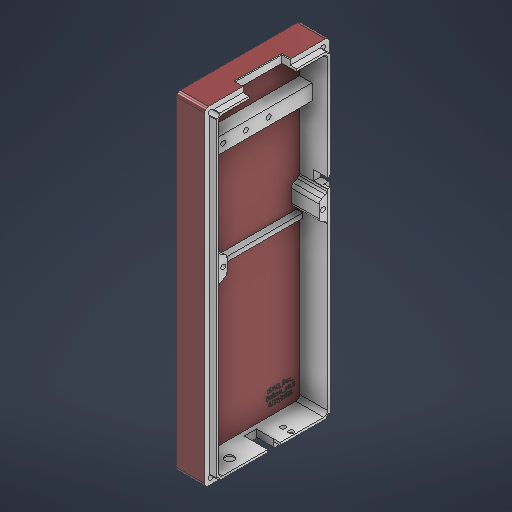
# Autodesk Inventor part: cDAQ_Box_Bottom_v0.2
Saved by Autodesk Inventor 2027 (Build 310192000, 192)
## iProperties
Created: 2026-05-08
Part Number: cDAQ_Box_Bottom_v0.2
Material: Generic
Document SubType Name: Modeling
Designer: giese
Density: 1 g/cm^3
Appearance: Default
Author: giese
Autodesk Inventor part; units mm, degrees
(part 1 of 2)
ref_plane "YZ Plane" through (0, 0, 0) normal (1, 0, 0) x (0, 1, 0)
ref_plane "XZ Plane" through (0, 0, 0) normal (0, 1, 0) x (-1, 0, 0)
ref_plane "XY Plane" through (0, 0, 0) normal (0, 0, 1) x (1, 0, 0)
sketch "Sketch1" plane through (0, 0, 0) normal (1, 0, 0) x (0, 1, 0)
  line L0 (37.5698, 53.1667) -> (-230.1462, 53.1667)
  line L1 (-230.1462, 53.1667) -> (-230.1462, -48.4333)
  line L2 (-230.1462, -48.4333) -> (37.5698, -48.4333)
  line L3 (37.5698, -48.4333) -> (37.5698, 53.1667)
  point P0 (0, 0)
  dimension "d0" = 101.6
  dimension "d1" = 267.716
  constraints: 8 end point, 2 parallel, 1 horizontal, 1 perpendicular
  measures "d0" distance of L2.end L0.start
  measures "d1" distance of L1.end L2.end
extrude "Extrusion1" add sketch "Sketch1" along normal blind 22.86
sketch "Sketch2" plane through (22.86, 0, 0) normal (1, 0, 0) x (0, 0, -1)
  line L0 (42.0833, 31.2198) -> (-46.8167, 31.2198)
  line L1 (-46.8167, 31.2198) -> (-46.8167, -223.7962)
  line L2 (-46.8167, -223.7962) -> (42.0833, -223.7962)
  line L3 (42.0833, -223.7962) -> (42.0833, 31.2198)
  line L4 (48.4333, 37.5698) -> (-53.1667, 37.5698) projected
  line L5 (-53.1667, 37.5698) -> (-53.1667, -230.1462) projected
  line L6 (-53.1667, -230.1462) -> (48.4333, -230.1462) projected
  point P0 (0, 0)
  dimension "d4" = 255.016
  dimension "d5" = 88.9
  dimension "d8" = 6.35
  dimension "d21" = 6.35
  dimension "d690" = 6.35
  constraints: 8 end point, 2 parallel, 1 horizontal, 1 perpendicular
  measures "d4" distance of L2.end L0.start
  measures "d5" distance of L0.start L0.end
  measures "d8" distance between parallel lines of L0 L4
  measures "d21" distance between parallel lines of L5 L1
  measures "d690" distance between parallel lines of L6 L2
extrude "Extrusion2" cut sketch "Sketch2" against normal blind 17.78
sketch "Sketch3" plane through (0, 0, 0) normal (-1, 0, 0) x (0, 0, 1)
  circle A0 centre (-6.6909, -2.0542) radius 2
  circle A1 centre (11.8079, -2.0542) radius 2
  circle A2 centre (30.3067, -2.0542) radius 2
  line L0 (-48.4333, -230.1462) -> (-48.4333, 37.5698) projected
  line L1 (-48.4333, 37.5698) -> (53.1667, 37.5698) projected
  line L2 (53.1667, 37.5698) -> (53.1667, -230.1462) projected
  line L3 (46.8167, 31.2198) -> (-42.0833, 31.2198) projected
  point P0 (0, 0)
  point P1 (-0.896, -23.7433)
  point P2 (-45.1848, 27.0137)
  dimension "d9" = 18.4988
  dimension "d10" = 4
  dimension "d11" = 4
  dimension "d12" = 18.4988
  dimension "d13" = 36.9976
  dimension "d18" = 22.86
  dimension "d22" = 4
  dimension "d58" = 39.624
  constraints: 3 centre point
  measures "d9" distance of A0.centre A1.centre
  measures "d10" diameter of A1
  measures "d11" diameter of A2
  measures "d12" distance of A1.centre A2.centre
  measures "d13" distance of A0.centre A2.centre
  measures "d18" distance from line of L2 A2.centre
  measures "d22" diameter of A0
  measures "d58" distance from line of L1 A2.centre
extrude "Extrusion3" cut sketch "Sketch3" against normal blind 5.08
sketch "Sketch5" plane through (0, -230.1462, -48.4333) normal (0, 0, -1) x (-1, 0, 0)
  line L0 (-27.2034, 165.862) -> (-16.51, 165.862)
  line L1 (-16.51, 165.862) -> (-16.51, 173.862)
  line L2 (-16.51, 173.862) -> (-27.2034, 173.862)
  line L3 (-27.2034, 173.862) -> (-27.2034, 165.862)
  line L4 (0, 267.716) -> (-22.86, 267.716) projected
  line L5 (0, 0) -> (0, 267.716) projected
  line L6 (-22.86, 0) -> (-22.86, 267.716) projected
  point P0 (0, 230.1462)
  point P1 (-21.8567, 173.862)
  point P2 (-21.8567, 165.862)
  dimension "d28" = 10.6934
  dimension "d30" = 8
  dimension "d31" = 16.51
  dimension "d34" = 101.854
  dimension "d215" = 4.3434
  constraints: 8 end point, 2 midpoint, 2 parallel, 1 horizontal, 1 perpendicular
  measures "d28" distance between parallel lines of L1 L3
  measures "d30" distance of point (-21.857, 173.862) point (-21.857, 165.862)
  measures "d31" distance between parallel lines of L5 L1
  measures "d34" distance between parallel lines of L4 L0
  measures "d215" distance between parallel lines of L6 L3
extrude "Extrusion4" cut sketch "Sketch5" against normal blind 24.13
sketch "Sketch6" plane through (0, -230.1462, -48.4333) normal (0, -1, 0) x (1, 0, 0)
  line L0 (24.08, 55.136) -> (16.08, 55.136)
  line L1 (16.08, 45.136) -> (24.08, 45.136)
  line L2 (0, 101.6) -> (0, 0) projected
  line L3 (28.36, 53.1359) -> (28.36, 47.136)
  line L4 (24.08, 55.136) -> (28.36, 53.1359)
  line L5 (28.36, 47.136) -> (24.08, 45.136)
  line L6 (0, 0) -> (22.86, 0) projected
  line L7 (22.86, 95.25) -> (22.86, 6.35) projected
  line L8 (22.86, 41.9134) -> (22.86, 37.4697)
  line L9 (16.08, 55.136) -> (8.636, 55.136)
  line L10 (8.636, 55.136) -> (8.636, 45.136)
  line L11 (8.636, 45.136) -> (21.16, 45.136)
  point P0 (0, 48.4333)
  point P1 (20.08, 55.136)
  point P2 (20.08, 45.136)
  point P3 (16.08, 50.136)
  dimension "d39" = 6
  dimension "d48" = 55.136
  dimension "d221" = 0
  dimension "d223" = 2
  dimension "d224" = 2
  dimension "d225" = 5.5
  dimension "d227" = 4.28
  dimension "d672" = 8.636
  constraints: 18 end point, 2 horizontal, 2 midpoint, 2 parallel, 2 point on line, 1 perpendicular, 1 vertical
  measures "d39" distance of L3.start L3.end
  measures "d48" distance between parallel lines of L6 L0
  measures "d221" horizontal distance of L0.start L1.end
  measures "d223" vertical distance of L3.end L1.end
  measures "d224" vertical distance of L0.start L3.start
  measures "d225" distance between parallel lines of L3 L7
  measures "d227" distance from line of L1.end L3
  measures "d672" distance between parallel lines of L2 L10
extrude "Extrusion5" cut sketch "Sketch6" against normal blind 6.35
sketch "Sketch7" plane through (0, 37.5698, 53.1667) normal (0, 1, 0) x (1, 0, 0)
  line L0 (31.0134, 69.85) -> (16.002, 69.85)
  line L1 (16.002, 69.85) -> (16.002, 31.75)
  line L2 (16.002, 31.75) -> (31.0134, 31.75)
  line L3 (31.0134, 31.75) -> (31.0134, 69.85)
  line L4 (0, 0) -> (22.86, 0) projected
  line L5 (0, 101.6) -> (0, 0) projected
  line L6 (22.86, 101.6) -> (22.86, 0) projected
  point P0 (0, 53.1667)
  point P1 (22.86, 69.85)
  point P2 (22.86, 31.75)
  dimension "d51" = 38.1
  dimension "d52" = 31.75
  dimension "d55" = 16.002
  dimension "d56" = 15.0114
  dimension "d57" = 8.1534
  constraints: 8 end point, 2 parallel, 1 horizontal, 1 perpendicular
  measures "d51" distance of L2.end L0.start
  measures "d52" distance between parallel lines of L4 L2
  measures "d55" distance between parallel lines of L5 L1
  measures "d56" distance between parallel lines of L3 L1
  measures "d57" distance between parallel lines of L6 L3
extrude "Extrusion6" cut sketch "Sketch7" against normal blind 7.62
fillet "Fillet1" radius 3.175 4 edges at (11.43, 37.5698, -48.4333) (11.43, 37.5698, 53.1667) (11.43, -230.1462, -48.4333) (11.43, -230.1462, 53.1667)
sketch "Sketch8" plane through (0, 0, 0) normal (-1, 0, 0) x (0, 0, 1)
  line L0 (-8.4625, -5.5848) -> (-4.9319, -5.5848)
  line L1 (-8.4625, 1.4764) -> (-4.9319, 1.4764)
  line L2 (-8.4625, -5.5848) -> (-10.5009, -2.0542)
  line L3 (-8.4625, 1.4764) -> (-10.5009, -2.0542)
  line L4 (-4.9319, -5.5848) -> (-2.8936, -2.0542)
  line L5 (-4.9319, 1.4764) -> (-2.8936, -2.0542)
  circle A0 centre (-6.6909, -2.0542) radius 2 projected
  line L6 (10.0363, -5.5848) -> (13.5669, -5.5848)
  line L7 (10.0363, 1.4764) -> (13.5669, 1.4764)
  line L8 (10.0363, -5.5848) -> (7.9979, -2.0542)
  line L9 (10.0363, 1.4764) -> (7.9979, -2.0542)
  line L10 (13.5669, -5.5848) -> (15.6053, -2.0542)
  line L11 (13.5669, 1.4764) -> (15.6053, -2.0542)
  circle A1 centre (11.8079, -2.0542) radius 2 projected
  line L12 (28.5351, -5.5848) -> (26.4967, -2.0542)
  line L13 (28.5351, 1.4764) -> (26.4967, -2.0542)
  line L14 (28.5351, -5.5848) -> (32.0657, -5.5848)
  line L15 (28.5351, 1.4764) -> (32.0657, 1.4764)
  line L16 (32.0657, -5.5848) -> (34.1041, -2.0542)
  line L17 (32.0657, 1.4764) -> (34.1041, -2.0542)
  circle A2 centre (30.3067, -2.0542) radius 2 projected
  point P0 (-6.6972, -5.5848)
  point P1 (11.8016, -5.5848)
  point P2 (30.3004, -5.5848)
  point P3 (-10.5009, -2.0542)
  point P4 (-2.8936, -2.0542)
  point P5 (15.6053, -2.0542)
  point P6 (7.9979, -2.0542)
  point P7 (34.1041, -2.0542)
  point P8 (26.4967, -2.0542)
  dimension "d60" = 7.0612
  dimension "d61" = 120
  dimension "d62" = 120
  dimension "d63" = 120
  dimension "d64" = 120
  dimension "d65" = 3.5306
  dimension "d66" = 3.5306
  dimension "d67" = 3.5306
  dimension "d68" = 3.5306
  dimension "d69" = 3.5306
  dimension "d70" = 3.5306
  dimension "d71" = 0
  dimension "d72" = 7.6074
  dimension "d73" = 3.81
  dimension "d74" = 0
  dimension "d75" = 7.0612
  dimension "d76" = 120
  dimension "d77" = 120
  dimension "d78" = 120
  dimension "d79" = 120
  dimension "d80" = 3.5306
  dimension "d81" = 3.5306
  dimension "d82" = 3.5306
  dimension "d83" = 3.5306
  dimension "d84" = 3.5306
  dimension "d85" = 3.5306
  dimension "d86" = 0
  dimension "d87" = 7.6074
  dimension "d91" = 0
  dimension "d92" = 3.81
  dimension "d93" = 7.0612
  dimension "d94" = 120
  dimension "d95" = 120
  dimension "d96" = 120
  dimension "d97" = 120
  dimension "d98" = 3.5306
  dimension "d99" = 3.5306
  dimension "d100" = 3.5306
  dimension "d101" = 3.5306
  dimension "d102" = 3.5306
  dimension "d103" = 3.5306
  dimension "d104" = 0
  dimension "d105" = 7.6074
  dimension "d108" = 0
  dimension "d109" = 3.81
  constraints: 36 end point, 6 horizontal, 3 midpoint
  measures "d60" distance from line of point (-6.697, -5.585) L1
  measures "d61" angle of L0 L2
  measures "d62" angle of L1 L3
  measures "d63" angle of L4 L0
  measures "d64" angle of L5 L1
  measures "d65" distance of L0.start L0.end
  measures "d66" distance of L1.start L1.end
  measures "d67" vertical distance of L1.start L3.end
  measures "d68" vertical distance of L0.start L2.end
  measures "d69" vertical distance of L1.end L5.end
  measures "d70" vertical distance of L0.end L4.end
  measures "d71" horizontal distance of L0.start L1.start
  measures "d72" distance of L4.end L2.end
  measures "d73" distance of A0.centre L2.end
  measures "d74" vertical distance of A0.centre L4.end
  measures "d75" distance from line of point (11.802, -5.585) L7
  measures "d76" angle of L6 L8
  measures "d77" angle of L7 L9
  measures "d78" angle of L10 L6
  measures "d79" angle of L11 L7
  measures "d80" distance of L8.start L6.end
  measures "d81" distance of L9.start L7.end
  measures "d82" vertical distance of L9.start L9.end
  measures "d83" vertical distance of L8.start L8.end
  measures "d84" vertical distance of L7.end L11.end
  measures "d85" vertical distance of L6.end L10.end
  measures "d86" horizontal distance of L8.start L9.start
  measures "d87" distance of L10.end L8.end
  measures "d91" vertical distance of A1.centre L8.end
  measures "d92" distance of A1.centre L8.end
  measures "d93" distance from line of point (30.3, -5.585) L15
  measures "d94" angle of L14 L12
  measures "d95" angle of L15 L13
  measures "d96" angle of L16 L14
  measures "d97" angle of L17 L15
  measures "d98" distance of L12.start L16.start
  measures "d99" distance of L15.start L15.end
  measures "d100" vertical distance of L15.start L13.end
  measures "d101" vertical distance of L12.start L12.end
  measures "d102" vertical distance of L15.end L17.end
  measures "d103" vertical distance of L16.start L16.end
  measures "d104" horizontal distance of L12.start L15.start
  measures "d105" distance of L16.end L12.end
  measures "d108" vertical distance of A2.centre L12.end
  measures "d109" distance of A2.centre L12.end
extrude "Extrusion7" cut sketch "Sketch8" against normal blind 4 contours L2 L3 L1 L5 L4 L0 | A0 | L8 L9 L7 L11 L10 L6 | A1 | L12 L13 L15 L17 L16 L14 | A2
sketch "Sketch9" plane through (5.08, 0, 0) normal (1, 0, 0) x (0, 0, -1)
  arc A0 (24.8089, -180.8044) -> (19.3527, -180.8044) centre (22.0808, -178.3302) ccw
  line L0 (45.2583, 37.5698) -> (16.6833, 37.5698) projected
  line L1 (42.0833, 31.2198) -> (42.0833, -223.7962) projected
  arc A1 (20.1758, -185.9502) -> (23.9858, -185.9502) centre (22.0808, -185.9502) ccw
  line L2 (23.9858, -185.9502) -> (23.9858, -182.9374)
  line L3 (20.1758, -185.9502) -> (20.1758, -182.9374)
  arc A2 (24.8089, -180.8044) -> (23.9858, -182.9374) centre (27.1608, -182.9374) ccw
  arc A3 (20.1758, -182.9374) -> (19.3527, -180.8044) centre (17.0008, -182.9374) ccw
  arc A4 (-25.9911, -180.8044) -> (-31.4473, -180.8045) centre (-28.7192, -178.3302) ccw
  arc A5 (-30.6242, -185.9366) -> (-26.8142, -185.9502) centre (-28.7192, -185.9502) ccw
  line L4 (-26.8142, -185.9502) -> (-26.8142, -182.9374)
  line L5 (-30.6242, -185.9366) -> (-30.6242, -182.9374)
  arc A6 (-25.9911, -180.8044) -> (-26.8142, -182.9374) centre (-23.6392, -182.9374) ccw
  arc A7 (-30.6242, -182.9374) -> (-31.4473, -180.8045) centre (-33.7992, -182.9374) ccw
  line L6 (-21.4167, 37.5698) -> (-49.9917, 37.5698) projected
  line L7 (-46.8167, -223.7962) -> (-46.8167, 31.2198) projected
  point P0 (0, 0)
  point P1 (23.9858, -181.4823)
  point P2 (20.1758, -181.4823)
  point P3 (-26.8142, -181.4823)
  point P4 (-30.6242, -181.4823)
  dimension "d112" = 215.9
  dimension "d114" = 7.366
  dimension "d116" = 3.81
  dimension "d117" = 223.52
  dimension "d118" = 3.175
  dimension "d119" = 7.366
  dimension "d120" = 3.81
  dimension "d121" = 3.175
  dimension "d122" = 215.9
  dimension "d123" = 223.52
  dimension "d125" = 0
  dimension "d128" = 50.8
  dimension "d129" = 20.0025
  dimension "d130" = 0
  constraints: 20 point on circle, 8 centre point, 8 end point, 8 tangent, 4 point on line, 2 equal radius, 2 parallel, 2 vertical
  measures "d112" distance from line of L0 A0.centre
  measures "d114" diameter of A0
  measures "d116" diameter of A1
  measures "d117" distance from line of L0 A1.centre
  measures "d118" radius of A2
  measures "d119" diameter of A4
  measures "d120" diameter of A5
  measures "d121" radius of A6
  measures "d122" distance from line of A4.centre L6
  measures "d123" distance from line of L6 A5.centre
  measures "d125" horizontal distance of A5.centre A4.centre
  measures "d128" distance of A5.centre A1.centre
  measures "d129" distance from line of L1 A0.centre
  measures "d130" horizontal distance of A0.centre A1.centre
extrude "Extrusion8" [suppressed]
sketch "Sketch10" plane through (22.86, 0, 0) normal (1, 0, 0) x (0, 0, -1)
  line L0 (-46.8167, 31.2198) -> (42.0833, 31.2198) projected
  line L1 (-46.8167, 31.2198) -> (42.0833, 31.2198)
  line L2 (42.0833, 33.2264) -> (-46.8167, 33.2264)
  line L3 (-46.8167, 33.2264) -> (-48.8233, 33.2264)
  line L4 (-48.8233, 33.2264) -> (-48.8233, -225.8028)
  line L5 (-48.8233, -225.8028) -> (44.0899, -225.8028)
  line L6 (44.0899, -225.8028) -> (44.0899, 33.2264)
  line L7 (44.0899, 33.2264) -> (41.9392, 33.2264)
  line L8 (42.0833, 31.2198) -> (42.0833, -223.7962) projected
  line L9 (-46.8167, -223.7962) -> (-46.8167, 31.2198) projected
  line L10 (42.0833, -223.7962) -> (-46.8167, -223.7962) projected
  line L11 (45.2583, 37.5698) -> (16.6833, 37.5698) projected
  dimension "d202" = 2.0066
  dimension "d203" = 2.0066
  dimension "d204" = 2.0066
  dimension "d205" = 2.0066
  dimension "d208" = 4.3434
  constraints: 14 end point, 3 perpendicular, 3 point on line, 1 collinear, 1 horizontal
  measures "d202" distance between parallel lines of L0 L2
  measures "d203" distance between parallel lines of L6 L8
  measures "d204" distance between parallel lines of L4 L9
  measures "d205" distance between parallel lines of L5 L10
  measures "d208" distance between parallel lines of L11 L2
extrude "Extrusion9" add sketch "Sketch10" along normal blind 5
fillet "Fillet2" radius 3.175 8 edges at (16.47, 31.2198, -42.0833) (16.47, 31.2198, 46.8167) (16.47, -223.7962, 46.8167) (16.47, -223.7962, -42.0833) (25.36, 33.2264, -44.0899) (25.36, 33.2264, 48.8233) (25.36, -225.8028, -44.0899) (25.36, -225.8028, 48.8233)
sketch "Sketch13" plane through (27.86, 0, 0) normal (1, 0, 0) x (0, 0, -1)
  arc A0 (44.0833, 30.0448) -> (40.9083, 33.2198) centre (40.9083, 30.0448) ccw projected
  arc A1 (-45.6417, 33.2198) -> (-48.8167, 30.0448) centre (-45.6417, 30.0448) ccw projected
  arc A2 (40.9083, -212.0802) -> (44.0833, -208.9052) centre (40.9083, -208.9052) ccw projected
  arc A3 (-48.8167, -208.9052) -> (-45.6417, -212.0802) centre (-45.6417, -208.9052) ccw projected
  line L0 (-21.4167, 37.5698) -> (-49.9917, 37.5698) projected
  line L1 (-53.1667, 34.3948) -> (-53.1667, -226.9712) projected
  line L2 (-49.9917, -230.1462) -> (45.2583, -230.1462) projected
  arc A4 (-48.8167, -208.9052) -> (-45.6417, -212.0802) centre (-45.6417, -208.9052) ccw projected
  circle A5 centre (-48.0867, -225.0662) radius 1.9939
  circle A6 centre (43.3533, -225.0662) radius 1.9939
  line L3 (48.4333, -226.9712) -> (48.4333, 34.3948) projected
  circle A7 centre (43.3533, 32.4898) radius 1.9939
  line L4 (45.2583, 37.5698) -> (16.6833, 37.5698) projected
  circle A8 centre (-48.0867, 32.4898) radius 1.9939
  arc A9 (41.4904, -28.6131) -> (38.3154, -25.4381) centre (38.3154, -28.6131) ccw
  circle A10 centre (38.2733, -76.7302) radius 1.9939
  circle A11 centre (-43.0067, -76.7302) radius 1.9939
  point P0 (0, 0)
  point P1 (-47.8868, 32.2898)
  point P2 (-47.8868, -211.1503)
  point P3 (-47.8868, -211.1503)
  point P4 (45.8404, -24.2631)
  point P5 (42.6654, -21.0881)
  dimension "d405" = 120
  dimension "d178" = 5.08
  dimension "d179" = 5.08
  dimension "d180" = 3.9878
  dimension "d181" = 5.08
  dimension "d182" = 5.08
  dimension "d183" = 3.9878
  dimension "d184" = 3.9878
  dimension "d185" = 5.08
  dimension "d186" = 5.08
  dimension "d187" = 3.9878
  dimension "d188" = 5.08
  dimension "d189" = 5.08
  dimension "d326" = 3.9878
  dimension "d327" = 10.16
  dimension "d328" = 114.3
  dimension "d329" = 3.9878
  dimension "d330" = 10.16
  dimension "d331" = 114.3
  constraints: 7 centre point, 5 point on circle
  measures "d178" distance from line of L1 A5.centre
  measures "d179" distance from line of L2 A5.centre
  measures "d180" diameter of A5
  measures "d181" distance from line of L2 A6.centre
  measures "d182" distance from line of L3 A6.centre
  measures "d183" diameter of A6
  measures "d184" diameter of A7
  measures "d185" distance from line of L3 A7.centre
  measures "d186" distance from line of L4 A7.centre
  measures "d187" diameter of A8
  measures "d188" distance from line of L0 A8.centre
  measures "d189" distance from line of L1 A8.centre
  measures "d326" diameter of A10
  measures "d327" distance from line of L3 A10.centre
  measures "d328" distance from line of A10.centre L4
  measures "d329" diameter of A11
  measures "d330" distance from line of L1 A11.centre
  measures "d331" distance from line of L0 A11.centre
extrude "Extrusion11" cut sketch "Sketch13" against normal blind 25.4
sketch "Sketch14" plane through (5.08, 0, 0) normal (1, 0, 0) x (0, 0, -1)
  line L0 (16.7951, -204.0653) -> (36.0118, -204.0653) construction
  line L1 (36.0118, -204.0653) -> (36.0118, -212.8579) construction
  line L2 (36.0118, -212.8579) -> (16.7951, -212.8579) construction
  line L3 (16.7951, -212.8579) -> (16.7951, -204.0653) construction
  spline S0 degree 2 poles (16.7333, -207.2294) (16.4962, -207.2294) (16.1034, -207.0837) (15.9627, -206.9355) knots 0 0 0 1 2 2 2
  spline S1 degree 2 poles (15.9627, -206.9355) (15.8219, -206.7897) (15.6663, -206.3402) (15.6663, -206.0388) knots 0 0 0 1 2 2 2
  spline S2 degree 2 poles (15.6663, -206.0388) (15.6663, -205.7375) (15.8268, -205.2978) (15.9627, -205.1496) knots 0 0 0 1 2 2 2
  spline S3 degree 2 poles (15.9627, -205.1496) (16.0985, -204.999) (16.5011, -204.8384) (16.7333, -204.8384) knots 0 0 0 1 2 2 2
  spline S4 degree 2 poles (16.7333, -204.8384) (16.921, -204.8384) (17.2718, -204.9446) (17.4076, -205.0138) knots 0 0 0 1 2 2 2
  line L4 (17.4076, -205.0138) -> (17.4076, -205.446)
  line L5 (17.4076, -205.446) -> (17.3854, -205.446)
  spline S5 degree 2 poles (17.3854, -205.446) (17.3434, -205.4115) (17.215, -205.3225) (17.1236, -205.2756) knots 0 0 0 1 2 2 2
  spline S6 degree 2 poles (17.1236, -205.2756) (17.0421, -205.2361) (16.8247, -205.1743) (16.7259, -205.1743) knots 0 0 0 1 2 2 2
  spline S7 degree 2 poles (16.7259, -205.1743) (16.427, -205.1743) (16.0639, -205.6263) (16.0639, -206.0388) knots 0 0 0 1 2 2 2
  spline S8 degree 2 poles (16.0639, -206.0388) (16.0639, -206.4414) (16.4147, -206.8935) (16.7259, -206.8935) knots 0 0 0 1 2 2 2
  spline S9 degree 2 poles (16.7259, -206.8935) (16.9136, -206.8935) (17.2545, -206.7378) (17.3854, -206.6168) knots 0 0 0 1 2 2 2
  line L6 (17.3854, -206.6168) -> (17.4076, -206.6168)
  line L7 (17.4076, -206.6168) -> (17.4076, -207.0491)
  spline S10 degree 2 poles (17.4076, -207.0491) (17.3508, -207.0762) (17.1779, -207.1528) (17.1087, -207.1701) knots 0 0 0 1 2 2 2
  spline S11 degree 2 poles (17.1087, -207.1701) (17.0099, -207.1997) (16.8543, -207.2294) (16.7333, -207.2294) knots 0 0 0 1 2 2 2
  spline S12 degree 2 poles (20.1913, -205.656) (20.1913, -206.0734) (19.8529, -206.7453) (19.5689, -206.933) knots 0 0 0 1 2 2 2
  spline S13 degree 2 poles (19.5689, -206.933) (19.3367, -207.0787) (18.86, -207.1775) (18.4895, -207.1775) knots 0 0 0 1 2 2 2
  line L8 (18.4895, -207.1775) -> (17.788, -207.1775)
  line L9 (17.788, -207.1775) -> (17.788, -204.1295)
  line L10 (17.788, -204.1295) -> (18.4821, -204.1295)
  spline S14 degree 2 poles (18.4821, -204.1295) (18.9119, -204.1295) (19.4009, -204.258) (19.5738, -204.3716) knots 0 0 0 1 2 2 2
  spline S15 degree 2 poles (19.5738, -204.3716) (19.8678, -204.5667) (20.1913, -205.2114) (20.1913, -205.656) knots 0 0 0 1 2 2 2
  spline S16 degree 2 poles (19.769, -205.651) (19.769, -205.3003) (19.5368, -204.8038) (19.3071, -204.663) knots 0 0 0 1 2 2 2
  spline S17 degree 2 poles (19.3071, -204.663) (19.144, -204.5667) (18.776, -204.4803) (18.5018, -204.4803) knots 0 0 0 1 2 2 2
  line L11 (18.5018, -204.4803) -> (18.1931, -204.4803)
  line L12 (18.1931, -204.4803) -> (18.1931, -206.8268)
  line L13 (18.1931, -206.8268) -> (18.5018, -206.8268)
  spline S18 degree 2 poles (18.5018, -206.8268) (18.7711, -206.8268) (19.1786, -206.7403) (19.3441, -206.6242) knots 0 0 0 1 2 2 2
  spline S19 degree 2 poles (19.3441, -206.6242) (19.5565, -206.481) (19.769, -206.0067) (19.769, -205.651) knots 0 0 0 1 2 2 2
  line L14 (20.3025, -207.1775) -> (21.33, -204.1295)
  line L15 (21.33, -204.1295) -> (21.8289, -204.1295)
  line L16 (21.8289, -204.1295) -> (22.8565, -207.1775)
  line L17 (22.8565, -207.1775) -> (22.4292, -207.1775)
  line L18 (22.4292, -207.1775) -> (22.1525, -206.3254)
  line L19 (22.1525, -206.3254) -> (20.9891, -206.3254)
  line L20 (20.9891, -206.3254) -> (20.7125, -207.1775)
  line L21 (20.7125, -207.1775) -> (20.3025, -207.1775)
  line L22 (22.0414, -205.9796) -> (21.5696, -204.5445)
  line L23 (21.5696, -204.5445) -> (21.1003, -205.9796)
  line L24 (21.1003, -205.9796) -> (22.0414, -205.9796)
  spline S20 degree 2 poles (25.6772, -207.9235) (25.5661, -207.9506) (25.324, -207.9803) (25.203, -207.9803) knots 0 0 0 1 2 2 2
  spline S21 degree 2 poles (25.203, -207.9803) (24.8597, -207.9803) (24.4323, -207.5974) (24.4126, -207.2417) knots 0 0 0 1 2 2 2
  spline S22 degree 2 poles (24.4126, -207.2417) (24.3854, -207.2417) (24.3385, -207.2417) (24.3187, -207.2417) knots 0 0 0 1 2 2 2
  spline S23 degree 2 poles (24.3187, -207.2417) (24.01, -207.2417) (23.5135, -207.0318) (23.3357, -206.8268) knots 0 0 0 1 2 2 2
  spline S24 degree 2 poles (23.3357, -206.8268) (23.1603, -206.6242) (22.9726, -206.0314) (22.9726, -205.656) knots 0 0 0 1 2 2 2
  spline S25 degree 2 poles (22.9726, -205.656) (22.9726, -205.2707) (23.1628, -204.6877) (23.3381, -204.4803) knots 0 0 0 1 2 2 2
  spline S26 degree 2 poles (23.3381, -204.4803) (23.516, -204.2752) (24.0124, -204.0653) (24.3187, -204.0653) knots 0 0 0 1 2 2 2
  spline S27 degree 2 poles (24.3187, -204.0653) (24.6299, -204.0653) (25.1289, -204.2827) (25.3018, -204.4803) knots 0 0 0 1 2 2 2
  spline S28 degree 2 poles (25.3018, -204.4803) (25.4747, -204.6803) (25.6674, -205.2756) (25.6674, -205.656) knots 0 0 0 1 2 2 2
  spline S29 degree 2 poles (25.6674, -205.656) (25.6674, -206.2488) (25.2055, -207.0194) (24.8028, -207.1553) knots 0 0 0 1 2 2 2
  spline S30 degree 2 poles (24.8028, -207.1553) (24.8127, -207.2689) (24.872, -207.4517) (24.9189, -207.5036) knots 0 0 0 1 2 2 2
  spline S31 degree 2 poles (24.9189, -207.5036) (24.9757, -207.5678) (25.1314, -207.6271) (25.2697, -207.6271) knots 0 0 0 1 2 2 2
  spline S32 degree 2 poles (25.2697, -207.6271) (25.3512, -207.6271) (25.5735, -207.5752) (25.6229, -207.5554) knots 0 0 0 1 2 2 2
  line L25 (25.6229, -207.5554) -> (25.6772, -207.5554)
  line L26 (25.6772, -207.5554) -> (25.6772, -207.9235)
  spline S33 degree 2 poles (25.245, -205.656) (25.245, -205.3522) (25.1141, -204.8853) (24.9955, -204.7322) knots 0 0 0 1 2 2 2
  spline S34 degree 2 poles (24.9955, -204.7322) (24.8745, -204.5741) (24.5336, -204.416) (24.3212, -204.416) knots 0 0 0 1 2 2 2
  spline S35 degree 2 poles (24.3212, -204.416) (24.1014, -204.416) (23.7704, -204.5692) (23.6444, -204.7322) knots 0 0 0 1 2 2 2
  spline S36 degree 2 poles (23.6444, -204.7322) (23.5234, -204.8878) (23.3949, -205.3596) (23.3949, -205.656) knots 0 0 0 1 2 2 2
  spline S37 degree 2 poles (23.3949, -205.656) (23.3949, -206.2562) (23.8988, -206.8959) (24.3212, -206.8959) knots 0 0 0 1 2 2 2
  spline S38 degree 2 poles (24.3212, -206.8959) (24.7436, -206.8959) (25.245, -206.2562) (25.245, -205.656) knots 0 0 0 1 2 2 2
  line L27 (28.1225, -207.7901) -> (25.7711, -207.7901)
  line L28 (25.7711, -207.7901) -> (25.7711, -207.5258)
  line L29 (25.7711, -207.5258) -> (28.1225, -207.5258)
  line L30 (28.1225, -207.5258) -> (28.1225, -207.7901)
  spline S39 degree 2 poles (30.4666, -206.2414) (30.4666, -206.4686) (30.2937, -206.8169) (30.1504, -206.9305) knots 0 0 0 1 2 2 2
  spline S40 degree 2 poles (30.1504, -206.9305) (29.9775, -207.0639) (29.5848, -207.1775) (29.2736, -207.1775) knots 0 0 0 1 2 2 2
  line L31 (29.2736, -207.1775) -> (28.3992, -207.1775)
  line L32 (28.3992, -207.1775) -> (28.3992, -204.1295)
  line L33 (28.3992, -204.1295) -> (29.2069, -204.1295)
  spline S41 degree 2 poles (29.2069, -204.1295) (29.5329, -204.1295) (29.859, -204.1715) (30.0072, -204.253) knots 0 0 0 1 2 2 2
  spline S42 degree 2 poles (30.0072, -204.253) (30.1727, -204.3395) (30.3233, -204.6235) (30.3233, -204.8162) knots 0 0 0 1 2 2 2
  spline S43 degree 2 poles (30.3233, -204.8162) (30.3233, -205.0311) (30.0961, -205.3719) (29.896, -205.4683) knots 0 0 0 1 2 2 2
  line L34 (29.896, -205.4683) -> (29.896, -205.4831)
  spline S44 degree 2 poles (29.896, -205.4831) (30.1677, -205.5572) (30.4666, -205.9499) (30.4666, -206.2414) knots 0 0 0 1 2 2 2
  spline S45 degree 2 poles (30.0442, -206.2587) (30.0442, -206.0858) (29.9454, -205.8635) (29.7972, -205.7844) knots 0 0 0 1 2 2 2
  spline S46 degree 2 poles (29.7972, -205.7844) (29.7009, -205.735) (29.4736, -205.7054) (29.2637, -205.7054) knots 0 0 0 1 2 2 2
  line L35 (29.2637, -205.7054) -> (28.8043, -205.7054)
  line L36 (28.8043, -205.7054) -> (28.8043, -206.8317)
  line L37 (28.8043, -206.8317) -> (29.1328, -206.8317)
  spline S47 degree 2 poles (29.1328, -206.8317) (29.3995, -206.8317) (29.7058, -206.7823) (29.8244, -206.7033) knots 0 0 0 1 2 2 2
  spline S48 degree 2 poles (29.8244, -206.7033) (29.938, -206.6218) (30.0442, -206.4192) (30.0442, -206.2587) knots 0 0 0 1 2 2 2
  spline S49 degree 2 poles (29.901, -204.873) (29.901, -204.7643) (29.8269, -204.6013) (29.7453, -204.5544) knots 0 0 0 1 2 2 2
  spline S50 degree 2 poles (29.7453, -204.5544) (29.6465, -204.5) (29.407, -204.4753) (29.1921, -204.4753) knots 0 0 0 1 2 2 2
  line L38 (29.1921, -204.4753) -> (28.8043, -204.4753)
  line L39 (28.8043, -204.4753) -> (28.8043, -205.367)
  line L40 (28.8043, -205.367) -> (29.2637, -205.367)
  spline S51 degree 2 poles (29.2637, -205.367) (29.4539, -205.367) (29.6342, -205.3275) (29.7305, -205.2657) knots 0 0 0 1 2 2 2
  spline S52 degree 2 poles (29.7305, -205.2657) (29.8244, -205.2064) (29.901, -205.0162) (29.901, -204.873) knots 0 0 0 1 2 2 2
  spline S53 degree 2 poles (32.7192, -206.0339) (32.7192, -206.6119) (32.1635, -207.2417) (31.6991, -207.2417) knots 0 0 0 1 2 2 2
  spline S54 degree 2 poles (31.6991, -207.2417) (31.2224, -207.2417) (30.6765, -206.5921) (30.6765, -206.0339) knots 0 0 0 1 2 2 2
  spline S55 degree 2 poles (30.6765, -206.0339) (30.6765, -205.4609) (31.2397, -204.8261) (31.6991, -204.8261) knots 0 0 0 1 2 2 2
  spline S56 degree 2 poles (31.6991, -204.8261) (32.1635, -204.8261) (32.7192, -205.4584) (32.7192, -206.0339) knots 0 0 0 1 2 2 2
  spline S57 degree 2 poles (32.3216, -206.0339) (32.3216, -205.5893) (31.998, -205.157) (31.6991, -205.157) knots 0 0 0 1 2 2 2
  spline S58 degree 2 poles (31.6991, -205.157) (31.4003, -205.157) (31.0742, -205.5893) (31.0742, -206.0339) knots 0 0 0 1 2 2 2
  spline S59 degree 2 poles (31.0742, -206.0339) (31.0742, -206.4661) (31.4003, -206.9108) (31.6991, -206.9108) knots 0 0 0 1 2 2 2
  spline S60 degree 2 poles (31.6991, -206.9108) (31.9955, -206.9108) (32.3216, -206.4736) (32.3216, -206.0339) knots 0 0 0 1 2 2 2
  line L41 (34.8904, -207.1775) -> (34.4186, -207.1775)
  line L42 (34.4186, -207.1775) -> (33.8629, -206.3179)
  line L43 (33.8629, -206.3179) -> (33.2923, -207.1775)
  line L44 (33.2923, -207.1775) -> (32.8551, -207.1775)
  line L45 (32.8551, -207.1775) -> (33.648, -206.0438)
  line L46 (33.648, -206.0438) -> (32.8625, -204.8903)
  line L47 (32.8625, -204.8903) -> (33.3343, -204.8903)
  line L48 (33.3343, -204.8903) -> (33.8876, -205.7424)
  line L49 (33.8876, -205.7424) -> (34.4532, -204.8903)
  line L50 (34.4532, -204.8903) -> (34.8904, -204.8903)
  line L51 (34.8904, -204.8903) -> (34.1025, -206.0191)
  line L52 (34.1025, -206.0191) -> (34.8904, -207.1775)
  line L53 (37.2295, -207.7901) -> (34.878, -207.7901)
  line L54 (34.878, -207.7901) -> (34.878, -207.5258)
  line L55 (34.878, -207.5258) -> (37.2295, -207.5258)
  line L56 (37.2295, -207.5258) -> (37.2295, -207.7901)
  spline S61 degree 2 poles (16.9976, -211.2598) (16.9976, -211.4871) (16.8247, -211.8353) (16.6814, -211.949) knots 0 0 0 1 2 2 2
  spline S62 degree 2 poles (16.6814, -211.949) (16.5085, -212.0823) (16.1158, -212.196) (15.8046, -212.196) knots 0 0 0 1 2 2 2
  line L57 (15.8046, -212.196) -> (14.9302, -212.196)
  line L58 (14.9302, -212.196) -> (14.9302, -209.148)
  line L59 (14.9302, -209.148) -> (15.7379, -209.148)
  spline S63 degree 2 poles (15.7379, -209.148) (16.0639, -209.148) (16.39, -209.19) (16.5382, -209.2715) knots 0 0 0 1 2 2 2
  spline S64 degree 2 poles (16.5382, -209.2715) (16.7037, -209.3579) (16.8543, -209.642) (16.8543, -209.8346) knots 0 0 0 1 2 2 2
  spline S65 degree 2 poles (16.8543, -209.8346) (16.8543, -210.0495) (16.6271, -210.3904) (16.427, -210.4867) knots 0 0 0 1 2 2 2
  line L60 (16.427, -210.4867) -> (16.427, -210.5015)
  spline S66 degree 2 poles (16.427, -210.5015) (16.6987, -210.5756) (16.9976, -210.9684) (16.9976, -211.2598) knots 0 0 0 1 2 2 2
  spline S67 degree 2 poles (16.5752, -211.2771) (16.5752, -211.1042) (16.4764, -210.8819) (16.3282, -210.8029) knots 0 0 0 1 2 2 2
  spline S68 degree 2 poles (16.3282, -210.8029) (16.2319, -210.7535) (16.0046, -210.7238) (15.7947, -210.7238) knots 0 0 0 1 2 2 2
  line L61 (15.7947, -210.7238) -> (15.3353, -210.7238)
  line L62 (15.3353, -210.7238) -> (15.3353, -211.8502)
  line L63 (15.3353, -211.8502) -> (15.6638, -211.8502)
  spline S69 degree 2 poles (15.6638, -211.8502) (15.9305, -211.8502) (16.2368, -211.8008) (16.3554, -211.7217) knots 0 0 0 1 2 2 2
  spline S70 degree 2 poles (16.3554, -211.7217) (16.469, -211.6402) (16.5752, -211.4377) (16.5752, -211.2771) knots 0 0 0 1 2 2 2
  spline S71 degree 2 poles (16.432, -209.8914) (16.432, -209.7828) (16.3579, -209.6197) (16.2764, -209.5728) knots 0 0 0 1 2 2 2
  spline S72 degree 2 poles (16.2764, -209.5728) (16.1775, -209.5185) (15.938, -209.4938) (15.7231, -209.4938) knots 0 0 0 1 2 2 2
  line L64 (15.7231, -209.4938) -> (15.3353, -209.4938)
  line L65 (15.3353, -209.4938) -> (15.3353, -210.3854)
  line L66 (15.3353, -210.3854) -> (15.7947, -210.3854)
  spline S73 degree 2 poles (15.7947, -210.3854) (15.9849, -210.3854) (16.1652, -210.3459) (16.2615, -210.2842) knots 0 0 0 1 2 2 2
  spline S74 degree 2 poles (16.2615, -210.2842) (16.3554, -210.2249) (16.432, -210.0347) (16.432, -209.8914) knots 0 0 0 1 2 2 2
  spline S75 degree 2 poles (19.2503, -211.0523) (19.2503, -211.6303) (18.6945, -212.2602) (18.2301, -212.2602) knots 0 0 0 1 2 2 2
  spline S76 degree 2 poles (18.2301, -212.2602) (17.7534, -212.2602) (17.2075, -211.6106) (17.2075, -211.0523) knots 0 0 0 1 2 2 2
  spline S77 degree 2 poles (17.2075, -211.0523) (17.2075, -210.4793) (17.7707, -209.8445) (18.2301, -209.8445) knots 0 0 0 1 2 2 2
  spline S78 degree 2 poles (18.2301, -209.8445) (18.6945, -209.8445) (19.2503, -210.4768) (19.2503, -211.0523) knots 0 0 0 1 2 2 2
  spline S79 degree 2 poles (18.8526, -211.0523) (18.8526, -210.6077) (18.529, -210.1755) (18.2301, -210.1755) knots 0 0 0 1 2 2 2
  spline S80 degree 2 poles (18.2301, -210.1755) (17.9313, -210.1755) (17.6052, -210.6077) (17.6052, -211.0523) knots 0 0 0 1 2 2 2
  spline S81 degree 2 poles (17.6052, -211.0523) (17.6052, -211.4846) (17.9313, -211.9292) (18.2301, -211.9292) knots 0 0 0 1 2 2 2
  spline S82 degree 2 poles (18.2301, -211.9292) (18.5265, -211.9292) (18.8526, -211.492) (18.8526, -211.0523) knots 0 0 0 1 2 2 2
  spline S83 degree 2 poles (20.3371, -212.2404) (20.0234, -212.2404) (19.6702, -211.8823) (19.6702, -211.4945) knots 0 0 0 1 2 2 2
  line L67 (19.6702, -211.4945) -> (19.6702, -210.2274)
  line L68 (19.6702, -210.2274) -> (19.4108, -210.2274)
  line L69 (19.4108, -210.2274) -> (19.4108, -209.9087)
  line L70 (19.4108, -209.9087) -> (19.6702, -209.9087)
  line L71 (19.6702, -209.9087) -> (19.6702, -209.2517)
  line L72 (19.6702, -209.2517) -> (20.0555, -209.2517)
  line L73 (20.0555, -209.2517) -> (20.0555, -209.9087)
  line L74 (20.0555, -209.9087) -> (20.7644, -209.9087)
  line L75 (20.7644, -209.9087) -> (20.7644, -210.2274)
  line L76 (20.7644, -210.2274) -> (20.0555, -210.2274)
  line L77 (20.0555, -210.2274) -> (20.0555, -211.3166)
  spline S84 degree 2 poles (20.0555, -211.3166) (20.0555, -211.4895) (20.0678, -211.6797) (20.1098, -211.7612) knots 0 0 0 1 2 2 2
  spline S85 degree 2 poles (20.1098, -211.7612) (20.1444, -211.8329) (20.3, -211.9045) (20.4334, -211.9045) knots 0 0 0 1 2 2 2
  spline S86 degree 2 poles (20.4334, -211.9045) (20.5272, -211.9045) (20.7026, -211.8477) (20.7421, -211.8304) knots 0 0 0 1 2 2 2
  line L78 (20.7421, -211.8304) -> (20.7644, -211.8304)
  line L79 (20.7644, -211.8304) -> (20.7644, -212.1762)
  spline S87 degree 2 poles (20.7644, -212.1762) (20.6557, -212.2058) (20.4334, -212.2404) (20.3371, -212.2404) knots 0 0 0 1 2 2 2
  spline S88 degree 2 poles (21.74, -212.2404) (21.4263, -212.2404) (21.0731, -211.8823) (21.0731, -211.4945) knots 0 0 0 1 2 2 2
  line L80 (21.0731, -211.4945) -> (21.0731, -210.2274)
  line L81 (21.0731, -210.2274) -> (20.8138, -210.2274)
  line L82 (20.8138, -210.2274) -> (20.8138, -209.9087)
  line L83 (20.8138, -209.9087) -> (21.0731, -209.9087)
  line L84 (21.0731, -209.9087) -> (21.0731, -209.2517)
  line L85 (21.0731, -209.2517) -> (21.4584, -209.2517)
  line L86 (21.4584, -209.2517) -> (21.4584, -209.9087)
  line L87 (21.4584, -209.9087) -> (22.1673, -209.9087)
  line L88 (22.1673, -209.9087) -> (22.1673, -210.2274)
  line L89 (22.1673, -210.2274) -> (21.4584, -210.2274)
  line L90 (21.4584, -210.2274) -> (21.4584, -211.3166)
  spline S89 degree 2 poles (21.4584, -211.3166) (21.4584, -211.4895) (21.4708, -211.6797) (21.5128, -211.7612) knots 0 0 0 1 2 2 2
  spline S90 degree 2 poles (21.5128, -211.7612) (21.5474, -211.8329) (21.703, -211.9045) (21.8364, -211.9045) knots 0 0 0 1 2 2 2
  spline S91 degree 2 poles (21.8364, -211.9045) (21.9302, -211.9045) (22.1056, -211.8477) (22.1451, -211.8304) knots 0 0 0 1 2 2 2
  line L91 (22.1451, -211.8304) -> (22.1673, -211.8304)
  line L92 (22.1673, -211.8304) -> (22.1673, -212.1762)
  spline S92 degree 2 poles (22.1673, -212.1762) (22.0587, -212.2058) (21.8364, -212.2404) (21.74, -212.2404) knots 0 0 0 1 2 2 2
  spline S93 degree 2 poles (24.3311, -211.0523) (24.3311, -211.6303) (23.7753, -212.2602) (23.311, -212.2602) knots 0 0 0 1 2 2 2
  spline S94 degree 2 poles (23.311, -212.2602) (22.8342, -212.2602) (22.2884, -211.6106) (22.2884, -211.0523) knots 0 0 0 1 2 2 2
  spline S95 degree 2 poles (22.2884, -211.0523) (22.2884, -210.4793) (22.8515, -209.8445) (23.311, -209.8445) knots 0 0 0 1 2 2 2
  spline S96 degree 2 poles (23.311, -209.8445) (23.7753, -209.8445) (24.3311, -210.4768) (24.3311, -211.0523) knots 0 0 0 1 2 2 2
  spline S97 degree 2 poles (23.9334, -211.0523) (23.9334, -210.6077) (23.6098, -210.1755) (23.311, -210.1755) knots 0 0 0 1 2 2 2
  spline S98 degree 2 poles (23.311, -210.1755) (23.0121, -210.1755) (22.686, -210.6077) (22.686, -211.0523) knots 0 0 0 1 2 2 2
  spline S99 degree 2 poles (22.686, -211.0523) (22.686, -211.4846) (23.0121, -211.9292) (23.311, -211.9292) knots 0 0 0 1 2 2 2
  spline S100 degree 2 poles (23.311, -211.9292) (23.6074, -211.9292) (23.9334, -211.492) (23.9334, -211.0523) knots 0 0 0 1 2 2 2
  line L93 (27.3198, -212.196) -> (27.3198, -210.872)
  spline S101 degree 2 poles (27.3198, -210.872) (27.3198, -210.714) (27.2951, -210.4447) (27.2556, -210.3706) knots 0 0 0 1 2 2 2
  spline S102 degree 2 poles (27.2556, -210.3706) (27.2161, -210.2891) (27.0654, -210.2101) (26.9345, -210.2101) knots 0 0 0 1 2 2 2
  spline S103 degree 2 poles (26.9345, -210.2101) (26.8159, -210.2101) (26.5442, -210.3558) (26.4009, -210.4941) knots 0 0 0 1 2 2 2
  spline S104 degree 2 poles (26.4009, -210.4941) (26.4034, -210.5287) (26.4084, -210.625) (26.4084, -210.6893) knots 0 0 0 1 2 2 2
  line L94 (26.4084, -210.6893) -> (26.4084, -212.196)
  line L95 (26.4084, -212.196) -> (26.023, -212.196)
  line L96 (26.023, -212.196) -> (26.023, -210.872)
  spline S105 degree 2 poles (26.023, -210.872) (26.023, -210.714) (25.9983, -210.4447) (25.9588, -210.3706) knots 0 0 0 1 2 2 2
  spline S106 degree 2 poles (25.9588, -210.3706) (25.9193, -210.2891) (25.7686, -210.2101) (25.6377, -210.2101) knots 0 0 0 1 2 2 2
  spline S107 degree 2 poles (25.6377, -210.2101) (25.5142, -210.2101) (25.24, -210.3657) (25.1116, -210.4867) knots 0 0 0 1 2 2 2
  line L97 (25.1116, -210.4867) -> (25.1116, -212.196)
  line L98 (25.1116, -212.196) -> (24.7263, -212.196)
  line L99 (24.7263, -212.196) -> (24.7263, -209.9087)
  line L100 (24.7263, -209.9087) -> (25.1116, -209.9087)
  line L101 (25.1116, -209.9087) -> (25.1116, -210.1607)
  spline S108 degree 2 poles (25.1116, -210.1607) (25.2623, -210.01) (25.5587, -209.8445) (25.7365, -209.8445) knots 0 0 0 1 2 2 2
  spline S109 degree 2 poles (25.7365, -209.8445) (25.9391, -209.8445) (26.2527, -210.0298) (26.3343, -210.2397) knots 0 0 0 1 2 2 2
  spline S110 degree 2 poles (26.3343, -210.2397) (26.5096, -210.0446) (26.8406, -209.8445) (27.0333, -209.8445) knots 0 0 0 1 2 2 2
  spline S111 degree 2 poles (27.0333, -209.8445) (27.1815, -209.8445) (27.4235, -209.9359) (27.5125, -210.0396) knots 0 0 0 1 2 2 2
  spline S112 degree 2 poles (27.5125, -210.0396) (27.6038, -210.1434) (27.7051, -210.4546) (27.7051, -210.6893) knots 0 0 0 1 2 2 2
  line L102 (27.7051, -210.6893) -> (27.7051, -212.196)
  line L103 (27.7051, -212.196) -> (27.3198, -212.196)
  line L104 (30.2863, -212.8085) -> (27.9348, -212.8085)
  line L105 (27.9348, -212.8085) -> (27.9348, -212.5442)
  line L106 (27.9348, -212.5442) -> (30.2863, -212.5442)
  line L107 (30.2863, -212.5442) -> (30.2863, -212.8085)
  line L108 (32.329, -209.9087) -> (31.467, -212.196)
  line L109 (31.467, -212.196) -> (31.1211, -212.196)
  line L110 (31.1211, -212.196) -> (30.2665, -209.9087)
  line L111 (30.2665, -209.9087) -> (30.684, -209.9087)
  line L112 (30.684, -209.9087) -> (31.3089, -211.6699)
  line L113 (31.3089, -211.6699) -> (31.9288, -209.9087)
  line L114 (31.9288, -209.9087) -> (32.329, -209.9087)
  spline S113 degree 2 poles (34.4606, -210.672) (34.4606, -211.492) (33.9839, -212.2602) (33.4874, -212.2602) knots 0 0 0 1 2 2 2
  spline S114 degree 2 poles (33.4874, -212.2602) (32.9835, -212.2602) (32.5118, -211.4772) (32.5118, -210.6744) knots 0 0 0 1 2 2 2
  spline S115 degree 2 poles (32.5118, -210.6744) (32.5118, -209.8494) (32.9885, -209.0862) (33.4874, -209.0862) knots 0 0 0 1 2 2 2
  spline S116 degree 2 poles (33.4874, -209.0862) (33.9888, -209.0862) (34.4606, -209.8766) (34.4606, -210.672) knots 0 0 0 1 2 2 2
  spline S117 degree 2 poles (33.937, -211.6007) (33.9962, -211.45) (34.0456, -210.9857) (34.0456, -210.672) knots 0 0 0 1 2 2 2
  spline S118 degree 2 poles (34.0456, -210.672) (34.0456, -210.3583) (33.9962, -209.8964) (33.9345, -209.7408) knots 0 0 0 1 2 2 2
  spline S119 degree 2 poles (33.9345, -209.7408) (33.8727, -209.5852) (33.6579, -209.4246) (33.4874, -209.4246) knots 0 0 0 1 2 2 2
  spline S120 degree 2 poles (33.4874, -209.4246) (33.317, -209.4246) (33.0972, -209.5852) (33.0329, -209.7457) knots 0 0 0 1 2 2 2
  spline S121 degree 2 poles (33.0329, -209.7457) (32.9712, -209.9013) (32.9267, -210.3756) (32.9267, -210.6744) knots 0 0 0 1 2 2 2
  spline S122 degree 2 poles (32.9267, -210.6744) (32.9267, -210.9955) (32.9663, -211.4253) (33.0305, -211.5933) knots 0 0 0 1 2 2 2
  spline S123 degree 2 poles (33.0305, -211.5933) (33.0898, -211.7514) (33.3096, -211.9218) (33.4874, -211.9218) knots 0 0 0 1 2 2 2
  spline S124 degree 2 poles (33.4874, -211.9218) (33.6554, -211.9218) (33.8752, -211.7612) (33.937, -211.6007) knots 0 0 0 1 2 2 2
  line L115 (35.5054, -212.196) -> (35.0164, -212.196)
  line L116 (35.0164, -212.196) -> (35.0164, -211.613)
  line L117 (35.0164, -211.613) -> (35.5054, -211.613)
  line L118 (35.5054, -211.613) -> (35.5054, -212.196)
  line L119 (38.0001, -212.196) -> (36.1205, -212.196)
  line L120 (36.1205, -212.196) -> (36.1205, -211.7637)
  spline S125 degree 2 poles (36.1205, -211.7637) (36.323, -211.5735) (36.6836, -211.2203) (36.8565, -211.0301) knots 0 0 0 1 2 2 2
  spline S126 degree 2 poles (36.8565, -211.0301) (37.2048, -210.6473) (37.4592, -210.1878) (37.4592, -209.9433) knots 0 0 0 1 2 2 2
  spline S127 degree 2 poles (37.4592, -209.9433) (37.4592, -209.8149) (37.3802, -209.6222) (37.3085, -209.5605) knots 0 0 0 1 2 2 2
  spline S128 degree 2 poles (37.3085, -209.5605) (37.2369, -209.4987) (37.0492, -209.437) (36.9356, -209.437) knots 0 0 0 1 2 2 2
  spline S129 degree 2 poles (36.9356, -209.437) (36.8269, -209.437) (36.6046, -209.4913) (36.5033, -209.5333) knots 0 0 0 1 2 2 2
  spline S130 degree 2 poles (36.5033, -209.5333) (36.4169, -209.5679) (36.2563, -209.6667) (36.2069, -209.7012) knots 0 0 0 1 2 2 2
  line L121 (36.2069, -209.7012) -> (36.1847, -209.7012)
  line L122 (36.1847, -209.7012) -> (36.1847, -209.2665)
  spline S131 degree 2 poles (36.1847, -209.2665) (36.3107, -209.2048) (36.7627, -209.0837) (36.9652, -209.0837) knots 0 0 0 1 2 2 2
  spline S132 degree 2 poles (36.9652, -209.0837) (37.3925, -209.0837) (37.8742, -209.5358) (37.8742, -209.9211) knots 0 0 0 1 2 2 2
  spline S133 degree 2 poles (37.8742, -209.9211) (37.8742, -210.1014) (37.7902, -210.4027) (37.7161, -210.5312) knots 0 0 0 1 2 2 2
  spline S134 degree 2 poles (37.7161, -210.5312) (37.642, -210.6646) (37.4271, -210.9264) (37.3085, -211.0523) knots 0 0 0 1 2 2 2
  spline S135 degree 2 poles (37.3085, -211.0523) (37.1159, -211.2623) (36.6441, -211.7118) (36.5033, -211.8428) knots 0 0 0 1 2 2 2
  line L123 (36.5033, -211.8428) -> (38.0001, -211.8428)
  line L124 (38.0001, -211.8428) -> (38.0001, -212.196)
  spline S136 degree 2 poles (18.944, -216.2264) (18.944, -216.4611) (18.7884, -216.8587) (18.6574, -216.9921) knots 0 0 0 1 2 2 2
  spline S137 degree 2 poles (18.6574, -216.9921) (18.5216, -217.1329) (18.1807, -217.2786) (17.9757, -217.2786) knots 0 0 0 1 2 2 2
  spline S138 degree 2 poles (17.9757, -217.2786) (17.7707, -217.2786) (17.4323, -217.1403) (17.3039, -217.002) knots 0 0 0 1 2 2 2
  spline S139 degree 2 poles (17.3039, -217.002) (17.1458, -216.8365) (16.968, -216.2807) (16.968, -215.8757) knots 0 0 0 1 2 2 2
  spline S140 degree 2 poles (16.968, -215.8757) (16.968, -215.478) (17.131, -214.8383) (17.3014, -214.6011) knots 0 0 0 1 2 2 2
  spline S141 degree 2 poles (17.3014, -214.6011) (17.4669, -214.369) (17.9905, -214.1096) (18.3339, -214.1096) knots 0 0 0 1 2 2 2
  spline S142 degree 2 poles (18.3339, -214.1096) (18.4351, -214.1096) (18.613, -214.1294) (18.6797, -214.1516) knots 0 0 0 1 2 2 2
  line L125 (18.6797, -214.1516) -> (18.6797, -214.5443)
  line L126 (18.6797, -214.5443) -> (18.6624, -214.5443)
  spline S143 degree 2 poles (18.6624, -214.5443) (18.6056, -214.5147) (18.3981, -214.4628) (18.2795, -214.4628) knots 0 0 0 1 2 2 2
  spline S144 degree 2 poles (18.2795, -214.4628) (17.8992, -214.4628) (17.4323, -214.9766) (17.3879, -215.4805) knots 0 0 0 1 2 2 2
  spline S145 degree 2 poles (17.3879, -215.4805) (17.5336, -215.3792) (17.8399, -215.268) (18.0227, -215.268) knots 0 0 0 1 2 2 2
  spline S146 degree 2 poles (18.0227, -215.268) (18.2005, -215.268) (18.4673, -215.3397) (18.613, -215.4484) knots 0 0 0 1 2 2 2
  spline S147 degree 2 poles (18.613, -215.4484) (18.7809, -215.5743) (18.944, -215.9646) (18.944, -216.2264) knots 0 0 0 1 2 2 2
  spline S148 degree 2 poles (18.529, -216.2437) (18.529, -216.056) (18.4302, -215.8016) (18.3215, -215.7126) knots 0 0 0 1 2 2 2
  spline S149 degree 2 poles (18.3215, -215.7126) (18.24, -215.6484) (18.0375, -215.6064) (17.9313, -215.6064) knots 0 0 0 1 2 2 2
  spline S150 degree 2 poles (17.9313, -215.6064) (17.788, -215.6064) (17.5188, -215.6929) (17.3879, -215.7744) knots 0 0 0 1 2 2 2
  spline S151 degree 2 poles (17.3879, -215.7744) (17.3854, -215.8189) (17.3804, -215.9028) (17.3804, -215.9671) knots 0 0 0 1 2 2 2
  spline S152 degree 2 poles (17.3804, -215.9671) (17.3804, -216.2832) (17.5039, -216.671) (17.5978, -216.7723) knots 0 0 0 1 2 2 2
  spline S153 degree 2 poles (17.5978, -216.7723) (17.6843, -216.8686) (17.872, -216.9452) (17.9782, -216.9452) knots 0 0 0 1 2 2 2
  spline S154 degree 2 poles (17.9782, -216.9452) (18.2252, -216.9452) (18.529, -216.5944) (18.529, -216.2437) knots 0 0 0 1 2 2 2
  line L127 (20.5717, -214.0306) -> (19.3787, -217.8764)
  line L128 (19.3787, -217.8764) -> (19.0329, -217.8764)
  line L129 (19.0329, -217.8764) -> (20.221, -214.0306)
  line L130 (20.221, -214.0306) -> (20.5717, -214.0306)
  line L131 (22.6342, -217.2144) -> (21.1472, -217.2144)
  line L132 (21.1472, -217.2144) -> (21.1472, -216.9032)
  line L133 (21.1472, -216.9032) -> (21.7005, -216.9032)
  line L134 (21.7005, -216.9032) -> (21.7005, -214.8605)
  line L135 (21.7005, -214.8605) -> (21.1472, -214.8605)
  line L136 (21.1472, -214.8605) -> (21.1472, -214.5814)
  spline S155 degree 2 poles (21.1472, -214.5814) (21.4609, -214.5814) (21.7573, -214.4035) (21.7771, -214.1565) knots 0 0 0 1 2 2 2
  line L137 (21.7771, -214.1565) -> (22.0932, -214.1565)
  line L138 (22.0932, -214.1565) -> (22.0932, -216.9032)
  line L139 (22.0932, -216.9032) -> (22.6342, -216.9032)
  line L140 (22.6342, -216.9032) -> (22.6342, -217.2144)
  line L141 (25.1091, -214.6234) -> (23.7901, -217.2144)
  line L142 (23.7901, -217.2144) -> (23.3554, -217.2144)
  line L143 (23.3554, -217.2144) -> (24.7485, -214.5246)
  line L144 (24.7485, -214.5246) -> (23.1751, -214.5246)
  line L145 (23.1751, -214.5246) -> (23.1751, -214.1664)
  line L146 (23.1751, -214.1664) -> (25.1091, -214.1664)
  line L147 (25.1091, -214.1664) -> (25.1091, -214.6234)
  line L148 (26.7492, -214.0306) -> (25.5562, -217.8764)
  line L149 (25.5562, -217.8764) -> (25.2104, -217.8764)
  line L150 (25.2104, -217.8764) -> (26.3985, -214.0306)
  line L151 (26.3985, -214.0306) -> (26.7492, -214.0306)
  line L152 (28.9648, -217.2144) -> (27.0851, -217.2144)
  line L153 (27.0851, -217.2144) -> (27.0851, -216.7822)
  spline S156 degree 2 poles (27.0851, -216.7822) (27.2877, -216.592) (27.6483, -216.2388) (27.8212, -216.0486) knots 0 0 0 1 2 2 2
  spline S157 degree 2 poles (27.8212, -216.0486) (28.1695, -215.6657) (28.4239, -215.2063) (28.4239, -214.9618) knots 0 0 0 1 2 2 2
  spline S158 degree 2 poles (28.4239, -214.9618) (28.4239, -214.8333) (28.3449, -214.6407) (28.2732, -214.5789) knots 0 0 0 1 2 2 2
  spline S159 degree 2 poles (28.2732, -214.5789) (28.2016, -214.5172) (28.0139, -214.4554) (27.9002, -214.4554) knots 0 0 0 1 2 2 2
  spline S160 degree 2 poles (27.9002, -214.4554) (27.7916, -214.4554) (27.5693, -214.5097) (27.468, -214.5517) knots 0 0 0 1 2 2 2
  spline S161 degree 2 poles (27.468, -214.5517) (27.3815, -214.5863) (27.221, -214.6851) (27.1716, -214.7197) knots 0 0 0 1 2 2 2
  line L154 (27.1716, -214.7197) -> (27.1494, -214.7197)
  line L155 (27.1494, -214.7197) -> (27.1494, -214.285)
  spline S162 degree 2 poles (27.1494, -214.285) (27.2753, -214.2232) (27.7273, -214.1022) (27.9299, -214.1022) knots 0 0 0 1 2 2 2
  spline S163 degree 2 poles (27.9299, -214.1022) (28.3572, -214.1022) (28.8389, -214.5542) (28.8389, -214.9395) knots 0 0 0 1 2 2 2
  spline S164 degree 2 poles (28.8389, -214.9395) (28.8389, -215.1198) (28.7549, -215.4212) (28.6808, -215.5496) knots 0 0 0 1 2 2 2
  spline S165 degree 2 poles (28.6808, -215.5496) (28.6067, -215.683) (28.3918, -215.9448) (28.2732, -216.0708) knots 0 0 0 1 2 2 2
  spline S166 degree 2 poles (28.2732, -216.0708) (28.0806, -216.2807) (27.6088, -216.7303) (27.468, -216.8612) knots 0 0 0 1 2 2 2
  line L156 (27.468, -216.8612) -> (28.9648, -216.8612)
  line L157 (28.9648, -216.8612) -> (28.9648, -217.2144)
  spline S167 degree 2 poles (31.2693, -215.6904) (31.2693, -216.5105) (30.7926, -217.2786) (30.2962, -217.2786) knots 0 0 0 1 2 2 2